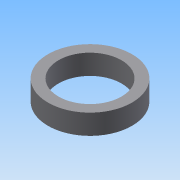
# Autodesk Inventor part: 主动轮锥齿轮配件
Saved by Autodesk Inventor 2015 (Build 190159000, 159)
## iProperties
Created: 2017-06-08
Part Number: 主动轮锥齿轮配件
Material: 铝 6061
Document SubType Name: Modeling
Designer: Administrator
Density: 2.7 g/cm^3
Appearance: 铝 - 平面
Author: Administrator
Autodesk Inventor part; units mm, degrees
ref_plane "YZ Plane" through (0, 0, 0) normal (1, 0, 0) x (0, 1, 0)
ref_plane "XZ Plane" through (0, 0, 0) normal (0, 1, 0) x (-1, 0, 0)
ref_plane "XY Plane" through (0, 0, 0) normal (0, 0, 1) x (1, 0, 0)
sketch "草图1" plane through (0, 0, 0) normal (0, 0, 1) x (1, 0, 0)
  circle A0 centre (0, 0) radius 20
  circle A1 centre (0, 0) radius 15
  dimension "d0" = 40
  dimension "d1" = 30
  constraints: 2 centre point, 2 coincident
  measures "d0" diameter of A0
  measures "d1" diameter of A1
extrude "拉伸1" add sketch "草图1" along normal blind 9.581
